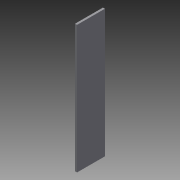
# Autodesk Inventor part: Front Paneling
Saved by Autodesk Inventor 2014 (Build 180170000, 170)
## iProperties
Created: 2014-01-21
Part Number: Front Paneling
Material: Generic
Document SubType Name: Modeling
Designer: NilesStanton
Density: 1 g/cm^3
Appearance: Default
Author: NilesStanton
Autodesk Inventor part; units mm, degrees
ref_plane "YZ Plane" through (0, 0, 0) normal (1, 0, 0) x (0, 1, 0)
ref_plane "XZ Plane" through (0, 0, 0) normal (0, 1, 0) x (-1, 0, 0)
ref_plane "XY Plane" through (0, 0, 0) normal (0, 0, 1) x (1, 0, 0)
sketch "Sketch1" plane through (0, 0, 0) normal (1, 0, 0) x (0, 1, 0)
  line L0 (-184.7273, 15.0091) -> (221.6727, 15.0091)
  line L1 (221.6727, 15.0091) -> (221.6727, -73.8909)
  line L2 (221.6727, -73.8909) -> (-184.7273, -73.8909)
  line L3 (-184.7273, -73.8909) -> (-184.7273, 15.0091)
  point P0 (0, 0)
  dimension "d0" = 406.4
  dimension "d2" = 88.9
  constraints: 8 end point, 2 parallel, 1 horizontal, 1 perpendicular
  measures "d0" distance of L1.end L2.end
  measures "d2" distance of L2.end L0.start
extrude "Extrusion1" add sketch "Sketch1" along normal blind 6.35
body "Solid1"
